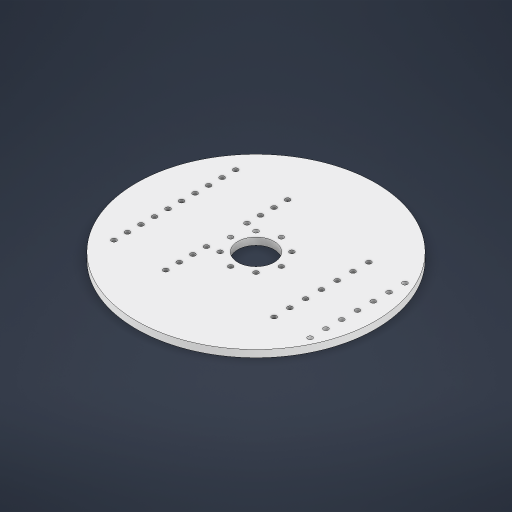
# Autodesk Inventor part: ArmBase
Saved by Autodesk Inventor 2024 (Build 280153000, 153)
## iProperties
Created: 2024-01-05
Part Number: ArmBase
Material: Aluminum 6061
Document SubType Name: Modeling
Designer: avsar
Density: 2.7 g/cm^3
Appearance: Aluminum - Flat
Author: avsar
Autodesk Inventor part; units mm, degrees
ref_plane "YZ Plane" through (0, 0, 0) normal (1, 0, 0) x (0, 1, 0)
ref_plane "XZ Plane" through (0, 0, 0) normal (0, 1, 0) x (-1, 0, 0)
ref_plane "XY Plane" through (0, 0, 0) normal (0, 0, 1) x (1, 0, 0)
sketch "Sketch1" plane through (0, 0, 0) normal (0, 1, 0) x (-1, 0, 0)
  circle A0 centre (0, 0) radius 106
  dimension "d1" = 212
  constraints: 1 centre point, 1 coincident
  measures "d1" diameter of A0
extrude "Extrusion1" add sketch "Sketch1" along normal mid plane 6.35
sketch "Sketch2" plane through (0, 3.175, 0) normal (0, 1, 0) x (1, 0, 0)
  circle A0 centre (0, 22.5) radius 2.05
  circle A1 centre (-15.9099, 15.9099) radius 2.05
  circle A2 centre (-22.5, 0) radius 2.05
  circle A3 centre (-15.9099, -15.9099) radius 2.05
  circle A4 centre (0, -22.5) radius 2.05
  circle A5 centre (15.9099, -15.9099) radius 2.05
  circle A6 centre (22.5, 0) radius 2.05
  circle A7 centre (15.9099, 15.9099) radius 2.05
  point P0 (0, 0)
  dimension "d4" = 4.1
  dimension "d5" = 22.5
  dimension "d8" = 360
  constraints: 8 centre point, 1 vertical alignment, 17 other
  measures "d4" diameter of A0
  measures "d5" distance of point (0, 0) A0.centre
extrude "Extrusion2" cut sketch "Sketch2" against normal through all
sketch "Sketch3" plane through (0, 3.175, 0) normal (0, 1, 0) x (1, 0, 0)
  circle A0 centre (0, 0) radius 16.1
  dimension "d12" = 32.2
  constraints: 1 centre point, 1 coincident
  measures "d12" diameter of A0
extrude "Extrusion3" cut sketch "Sketch3" against normal through all
sketch "Sketch8" plane through (0, 3.175, 0) normal (0, 1, 0) x (1, 0, 0)
  circle A0 centre (-26, -54) radius 2.1
  circle A1 centre (0, 0) radius 106 construction
  line L0 (0, -106) -> (0, 0) construction
  circle A2 centre (-26, -42) radius 2.1
  circle A3 centre (-26, -30) radius 2.1
  circle A4 centre (-26, -18) radius 2.1
  circle A5 centre (-26, -6) radius 2.1
  circle A6 centre (-26, 6) radius 2.1
  circle A7 centre (-26, 18) radius 2.1
  circle A8 centre (-26, 30) radius 2.1
  circle A9 centre (-26, 42) radius 2.1
  circle A10 centre (-26, 54) radius 2.1
  line L1 (-26, -6) -> (-26, 6) construction
  circle A11 centre (-72, -54) radius 2.1
  circle A12 centre (-72, -42) radius 2.1
  circle A13 centre (-72, -30) radius 2.1
  circle A14 centre (-72, -18) radius 2.1
  circle A15 centre (-72, -6) radius 2.1
  circle A16 centre (-72, 6) radius 2.1
  circle A17 centre (-72, 18) radius 2.1
  circle A18 centre (-72, 30) radius 2.1
  circle A19 centre (-72, 42) radius 2.1
  circle A20 centre (-72, 54) radius 2.1
  point P0 (-26, 0)
  dimension "d71" = 4.2
  dimension "d74" = 12
  dimension "d79" = 26
  dimension "d80" = 4.2
  dimension "d83" = 12
  dimension "d88" = 46
  constraints: 20 centre point, 4 end point, 4 vertical, 2 horizontal alignment, 1 midpoint, 1 vertical alignment, 37 other
  measures "d71" diameter of A0
  measures "d74" distance of A0.centre A2.centre
  measures "d79" distance of point (0, 0) point (-26, 0)
  measures "d80" diameter of A11
  measures "d83" distance of A11.centre A12.centre
  measures "d88" distance of A0.centre A11.centre
extrude "Extrusion7" cut sketch "Sketch8" against normal through all contours A0 | A2 | A3 | A4 | A7 | A8 | A9 | A10 | A11 | A12 | A13 | A14 | A15 | A16 | A17 | A18 | A19 | A20
sketch "Sketch9" plane through (0, 3.175, 0) normal (0, 1, 0) x (1, 0, 0)
  circle A0 centre (58, -42) radius 2.1
  line L0 (0, 0) -> (0, 16.1) construction
  circle A1 centre (0, 0) radius 16.1 construction
  line L1 (0, 0) -> (16.1, 0) construction
  circle A2 centre (58, -28) radius 2.1
  circle A3 centre (58, -14) radius 2.1
  circle A4 centre (58, 0) radius 2.1
  circle A5 centre (58, 14) radius 2.1
  circle A6 centre (58, 28) radius 2.1
  circle A7 centre (58, 42) radius 2.1
  circle A8 centre (90, -42) radius 2.1
  circle A9 centre (90, -28) radius 2.1
  circle A10 centre (90, -14) radius 2.1
  circle A11 centre (90, 0) radius 2.1
  circle A12 centre (90, 14) radius 2.1
  circle A13 centre (90, 28) radius 2.1
  circle A14 centre (90, 42) radius 2.1
  dimension "d91" = 4.2
  dimension "d92" = 58
  dimension "d93" = 42
  dimension "d96" = 14
  dimension "d99" = 32
  constraints: 14 centre point, 4 end point, 2 horizontal, 2 point on circle, 2 vertical, 26 other
  measures "d91" diameter of A0
  measures "d92" horizontal distance of L0.start A0.centre
  measures "d93" vertical distance of L0.start A0.centre
  measures "d96" distance of A0.centre A2.centre
  measures "d99" distance of A0.centre A8.centre
extrude "Extrusion8" cut sketch "Sketch9" against normal through all
body "Solid1"
